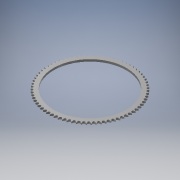
# Autodesk Inventor part: Roller Chain Sprocket2
Saved by Autodesk Inventor 2017 (Build 210142000, 142)
## iProperties
Created: 2016-10-04
Part Number: Roller Chain Sprocket2
Material: Steel
Document SubType Name: Modeling
Designer: hanso
Density: 1 g/cm^3
Appearance: Steel
CustomPartVersion: 1
Author: hanso
Autodesk Inventor part; units mm, degrees
ref_plane "YZ Plane" through (0, 0, 0) normal (1, 0, 0) x (0, 1, 0)
ref_plane "XZ Plane" through (0, 0, 0) normal (0, 1, 0) x (-1, 0, 0)
sketch "Theoretical Tooth Profile" plane through (0, 0, 0) normal (0, 0, 1) x (1, 0, 0)
  circle A0 centre (0, 0) radius 149.6188 construction
  line L0 (0, 0) -> (0, 149.6188) construction
  line L1 (0, 0) -> (12.6886, 149.0798) construction
  circle A1 centre (0, 0) radius 153.2939
  arc A2 (-3.2603, 147.2664) -> (3.2603, 147.2664) centre (0, 149.6188) ccw
  line L2 (0, 149.6188) -> (12.6886, 149.0798) construction
  line L3 (0, 149.6188) -> (5.1413, 153.3283) construction
  line L4 (5.1413, 153.3283) -> (-4.6796, 150.0294) construction
  arc A3 (6.1677, 153.1698) -> (5.0629, 151.1706) centre (11.0847, 149.1479) ccw
  arc A4 (-5.0629, 151.1706) -> (-6.1677, 153.1698) centre (-11.0847, 149.1479) ccw
  line L5 (-11.0847, 149.1479) -> (-5.0629, 151.1706) construction
  arc A5 (-4.6796, 150.0294) -> (-3.2603, 147.2664) centre (5.1413, 153.3283) ccw
  line L6 (-4.6796, 150.0294) -> (-5.0629, 151.1706)
  arc A6 (3.2603, 147.2664) -> (4.6796, 150.0294) centre (-5.1413, 153.3283) ccw
  line L7 (5.0629, 151.1706) -> (4.6796, 150.0294)
  line L8 (0, 0) -> (6.506, 153.1558) construction
  point P0 (6.3443, 149.3493)
  dimension "d0" = 299.2375
  dimension "d2" = 4.865
  dimension "d3" = 4.0203
  dimension "d10" = 125.811
  dimension "d11" = 17.243
  dimension "d12" = 6.3398
  dimension "d13" = 10.3602
  dimension "d14" = 11.0947
  dimension "d23" = 3.81
  constraints: 18 end point, 15 point on circle, 7 centre point, 3 coincident, 3 point on line, 3 symmetric about line, 3 tangent, 1 equal radius, 1 midpoint, 1 parallel, 1 vertical, 1 other
  measures "d0" diameter of A0
  measures "d2" angle of L1 L0
  measures "d3" radius of A2
  measures "d10" angle of L3 L0
  measures "d11" angle of L4 L3
  measures "d12" distance of L2.start L3.end
  measures "d13" distance of L3.end L4.end
  measures "d14" distance of A3.centre L0.end
  measures "d23" distance from line of L8.end L2
sketch "Tooth Profile" plane through (0, 0, 0) normal (0, 0, 1) x (1, 0, 0)
  circle A0 centre (0, 0) radius 153.2939 projected
  line L0 (0, 0) -> (0, 149.6188) construction
  line L1 (0, 149.6188) -> (3.7631, 148.2037) construction
  arc A1 (-3.7631, 148.2037) -> (3.7631, 148.2037) centre (0, 149.6188) ccw
  line L2 (-3.7631, 148.2037) -> (0, 149.6188) construction
  arc A2 (-3.7631, 148.2037) -> (-5.8506, 153.1823) centre (-71.4124, 122.7651) ccw
  arc A3 (5.8506, 153.1823) -> (3.7631, 148.2037) centre (71.4124, 122.7651) ccw
  dimension "d44" = 138.784
  dimension "d45" = 4.0203
  dimension "d46" = 72.2742
  constraints: 8 point on circle, 7 end point, 3 centre point, 2 tangent, 1 coincident, 1 equal radius, 1 symmetric about line, 1 vertical
  measures "d44" angle of L1 L2
  measures "d45" radius of A1
  measures "d46" radius of A3
sketch "Section Profile" plane through (0, 0, 0) normal (1, 0, 0) x (0, 1, 0)
  line L0 (153.2939, 0) -> (-153.2939, 0) projected
  line L1 (142.2449, 3.7612) -> (-142.2449, 3.7612)
  line L2 (-142.2449, 3.7612) -> (-142.2449, -3.7612)
  line L3 (-142.2449, -3.7612) -> (142.2449, -3.7612)
  line L4 (142.2449, -3.7612) -> (142.2449, 3.7612)
  line L5 (142.2449, 3.7612) -> (153.2939, 3.7612) construction
  line L6 (153.2939, 3.7612) -> (153.2939, -3.7612) construction
  line L7 (153.2939, -3.7612) -> (142.2449, -3.7612) construction
  line L8 (142.2449, -3.7612) -> (142.2449, 3.7612)
  arc A0 (153.2939, 2.1737) -> (146.9424, 3.7612) centre (146.9424, -9.7389) ccw
  arc A1 (146.9424, -3.7612) -> (153.2939, -2.1737) centre (146.9424, 9.7389) ccw
  line L9 (146.9424, 3.7612) -> (0, 3.7612)
  line L10 (0, 3.7612) -> (0, -3.7612)
  line L11 (0, -3.7612) -> (146.9424, -3.7612)
  line L12 (0, 3.7612) -> (0, -3.7612)
  line L13 (153.2939, 2.1737) -> (153.2939, -2.1737)
  point P0 (0, 0)
  point P1 (0, 0)
  dimension "d30" = 7.5225
  dimension "d31" = 284.4899
  dimension "d32" = 7.5225
  dimension "d33" = 1.5875
  dimension "d34" = 13.5001
  dimension "d43" = 3.7612
  constraints: 26 end point, 7 midpoint, 5 perpendicular, 4 parallel, 4 point on circle, 3 point on line, 3 symmetric about line, 2 centre point, 2 horizontal, 2 tangent, 1 collinear, 1 other
  measures "d30" distance between parallel lines of L7 L5
  measures "d31" distance between parallel lines of L2 L4
  measures "d32" distance between parallel lines of L3 L1
  measures "d33" distance from line of L13.start L5
  measures "d34" radius of A0
  measures "d43" distance between parallel lines of L3 L0
revolve "Shroud" add sketch "Section Profile" angle 360 about axis through (0, 0, 3.7612) along (0, 0, -1) contours L10 L3 L2 L0 | L0 L2 L1 L10
revolve "Strand" add sketch "Section Profile" angle 360 about axis through (0, 0, 3.7612) along (0, 0, -1) contours L13 A1 L11 L4 L0 | L0 L4 L9 A0 L13 | L4 L3 L10 L0 | L0 L10 L1 L4
pattern_of_one "Strand Pattern"
extrude "Theoretical Tooth" cut sketch "Theoretical Tooth Profile" along normal through all both and the other way through all contours A3 L7 A6 A2 A5 L6 A4 A1 picked at (0.6855, 149.271)
extrude "Tooth" [suppressed]
pattern_circular "Tooth Pattern" count 74 over 360 about axis through (0, 0, -10) along (0, 0, 1) of "Theoretical Tooth"
ref_plane "Timing Plane" through (0, 149.6188, 0) normal (1, 0, 0) x (0, 1, 0)
sketch "Sketch4" plane through (0, 149.6188, -3.7612) normal (0, 0, -1) x (-1, 0, 0)
  circle A0 centre (0, -149.6188) radius 132.2821
  constraints: 1 centre point, 1 coincident
extrude "Extrusion4" cut sketch "Sketch4" against normal blind 53.1
equation "\"d3\" = 0.5 * da_Dr + da_SC"
equation "\"d12\" = 0.8 * da_Dr"
equation "\"d13\" = 1.3 * da_Dr + da_SC"
equation "\"d14\" = 1.4 * da_Dr"
equation "\"d23\" = da_Ha"
equation "\"d44\" = da_Alfa"
equation "\"d45\" = da_Ri"
equation "\"d46\" = da_Re"
equation "\"d30\" = da_Bf"
equation "\"d31\" = da_Ds"
equation "\"d32\" = da_Bs"
equation "\"d33\" = da_Ba"
equation "\"d34\" = da_Rx"
equation "\"d40\" = da_pt"
equation "\"form_type\" = 0"
equation "\"da_p\" = 12.7"
equation "\"da_Dr\" = 7.9248"
equation "\"da_SC\" = 0.05791"
equation "\"da_Ha\" = 3.81"
equation "\"da_pt\" = 14.3764"
equation "\"da_Bf\" = 7.52246"
equation "\"da_Ba\" = 1.5875"
equation "\"da_Rx\" = 13.5001"
equation "\"da_Ra\" = 0.508"
equation "\"da_Bs\" = 7.52246"
equation "\"da_Ds\" = 284.48989"
equation "\"da_Re\" = 72.27418"
equation "\"da_Ri\" = 4.02031"
equation "\"da_Alfa\" = 138.784deg"
body "Solid1"
